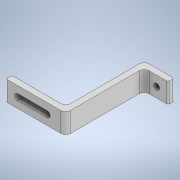
# Autodesk Inventor part: PowerBrick_Clamp
Saved by Autodesk Inventor 2021 (Build 250183000, 183)
## iProperties
Created: 2022-01-02
Part Number: PowerBrick_Clamp
Material: Generic
Document SubType Name: Modeling
Designer: Jorian Brusind
Density: 1 g/cm^3
Appearance: Default
Author: Jorian Brusind
Autodesk Inventor part; units mm, degrees
ref_plane "YZ Plane" through (0, 0, 0) normal (1, 0, 0) x (0, 1, 0)
ref_plane "XZ Plane" through (0, 0, 0) normal (0, 1, 0) x (-1, 0, 0)
ref_plane "XY Plane" through (0, 0, 0) normal (0, 0, 1) x (1, 0, 0)
sketch "Sketch1" plane through (0, 0, 0) normal (0, 1, 0) x (-1, 0, 0)
  line L0 (0, 0) -> (-60, 0)
  line L1 (-60, 0) -> (-60, -6)
  line L2 (-60, -6) -> (0, -6)
  line L3 (0, -6) -> (0, 0)
  line L4 (-60, 0) -> (-54, 0)
  line L5 (-54, 0) -> (-54, -85)
  line L6 (-54, -85) -> (-60, -85)
  line L7 (-60, -85) -> (-60, 0)
  line L8 (-54, -85) -> (-84, -85)
  line L9 (-84, -85) -> (-84, -79)
  line L10 (-84, -79) -> (-54, -79)
  line L11 (-54, -79) -> (-54, -85)
  point P0 (-60, -79)
  point P1 (-54, -6)
  dimension "d2" = 60
  dimension "d3" = 6
  dimension "d4" = 6
  dimension "d5" = 85
  dimension "d6" = 30
  dimension "d7" = 6
  constraints: 24 end point, 6 parallel, 3 horizontal, 3 perpendicular
  measures "d2" distance of L2.end L1.end
  measures "d3" distance of L1.end L0.end
  measures "d4" distance of L5.end L6.end
  measures "d5" distance of L4.end L5.end
  measures "d6" distance of L9.end L10.end
  measures "d7" distance of L8.end L9.end
extrude "Extrusion1" add sketch "Sketch1" along normal blind 20
fillet "Fillet1" radius 5 4 edges at (54, 10, -6) (60, 10, 0) (60, 10, -79) (54, 10, -85)
fillet "Fillet2" radius 1.5 4 edges at (0, 10, -6) (0, 10, 0) (84, 10, -85) (84, 10, -79)
sketch "Sketch2" plane through (49, 0, -6) normal (0, 0, -1) x (-1, 0, 0)
  line L0 (47.5, 0) -> (47.5, 20) projected
  line L1 (47.5, 10) -> (22.5, 10)
  line L2 (0, 0) -> (0, 20) projected
  line L3 (7.5, 10) -> (37.5, 10) construction
  line L4 (7.5, 7) -> (37.5, 7)
  line L5 (37.5, 13) -> (7.5, 13)
  arc A0 (7.5, 13) -> (7.5, 7) centre (7.5, 10) ccw
  arc A1 (37.5, 7) -> (37.5, 13) centre (37.5, 10) ccw
  point P0 (49, 0)
  dimension "d12" = 25
  dimension "d13" = 15
  dimension "d14" = 6
  constraints: 10 end point, 4 point on circle, 4 tangent, 2 centre point, 2 midpoint, 1 parallel, 1 perpendicular, 1 point on line
  measures "d12" distance of L1.start L1.end
  measures "d13" distance of L1.end L3.end
  measures "d14" diameter of A1
extrude "Extrusion2" cut sketch "Sketch2" against normal through all
sketch "Sketch3" plane through (59, 0, -85) normal (0, 0, -1) x (-1, 0, 0)
  line L0 (-23.5, 0) -> (-23.5, 20) projected
  line L1 (-23.5, 10) -> (-13.5, 10)
  line L2 (0, 20) -> (0, 0) projected
  circle A0 centre (-13.5, 10) radius 3
  point P0 (59, 0)
  dimension "d17" = 10
  dimension "d18" = 6
  constraints: 2 end point, 1 centre point, 1 coincident, 1 midpoint, 1 perpendicular
  measures "d17" distance of L1.start L1.end
  measures "d18" diameter of A0
extrude "Extrusion3" cut sketch "Sketch3" against normal through all
body "Solid1"
